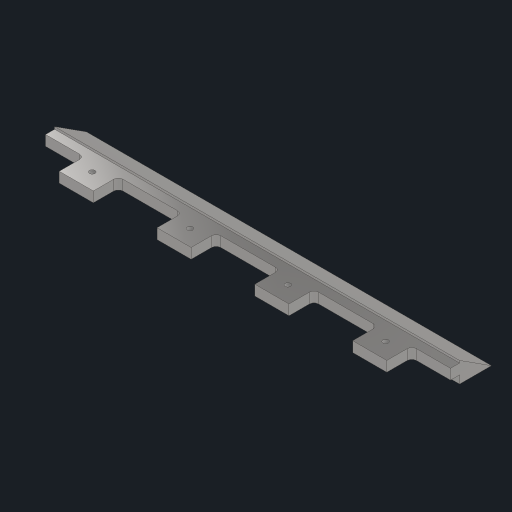
# Autodesk Inventor part: plog
Saved by Autodesk Inventor 2023 (Build 270158000, 158)
## iProperties
Created: 2024-04-10
Part Number: plog
Material: Steel, Alloy
Document SubType Name: Modeling
Designer: szymo
Density: 7.73 g/cm^3
Appearance: Semi-Polished
Mass: 132.729 g
Surface Area: 104.354 cm^2
Volume: 17.1707 cm^3
Author: szymo
Autodesk Inventor part; units mm, degrees
ref_plane "YZ Plane" through (0, 0, 0) normal (1, 0, 0) x (0, 1, 0)
ref_plane "XZ Plane" through (0, 0, 0) normal (0, 1, 0) x (-1, 0, 0)
ref_plane "XY Plane" through (0, 0, 0) normal (0, 0, 1) x (1, 0, 0)
sketch "Sketch3" plane through (0, 0, 0) normal (1, 0, 0) x (0, 1, 0)
  line L0 (0, 0) -> (9, 0)
  line L1 (9, 0) -> (9, -14)
  line L2 (9, -14) -> (0, -14)
  line L3 (0, -14) -> (0, 0)
  line L4 (9, 0) -> (0, -14)
  line L5 (8, 0) -> (3.5, 0)
  line L6 (3.5, 0) -> (3.5, 15)
  line L7 (3.5, 15) -> (8, 15)
  line L8 (8, 15) -> (8, 0)
  line L9 (8.5, 0) -> (8, 0)
  line L10 (8, 0) -> (8, 4)
  point P0 (3.5, 0)
  dimension "d30" = 15
  dimension "d31" = 4.5
  dimension "d63" = 9
  dimension "d141" = 32.735
  dimension "d142" = 14
  dimension "d143" = 3.5
  dimension "d144" = 1
  constraints: 22 end point, 4 perpendicular, 3 point on line, 1 collinear
  measures "d30" distance of L5.end L6.end
  measures "d31" distance of L6.end L7.end
  measures "d63" distance of L1.end L2.end
  measures "d141" angle of L4 L3
  measures "d142" distance of L0.end L1.end
  measures "d143" distance between parallel lines of L6 L3
  measures "d144" distance from line of L8 L0.end
extrude "Extrusion2" add sketch "Sketch3" along normal blind 178 contours L0 L4 L3 | L6 L7 L8 L0
sketch "Sketch10" plane through (0, 3.5, -14) normal (0, -1, 0) x (1, 0, 0)
  line L0 (0, 14) -> (0, 26)
  line L1 (0, 26) -> (178, 26)
  line L2 (178, 14) -> (178, 26)
  line L3 (0, 14) -> (0, 18)
  line L4 (0, 18) -> (17, 18)
  line L5 (17, 18) -> (17, 26)
  line L6 (17, 26) -> (0, 26)
  line L7 (0, 26) -> (0, 18)
  line L8 (0, 18) -> (178, 18)
  line L9 (178, 26) -> (161, 26)
  line L10 (161, 26) -> (161, 18)
  line L11 (161, 18) -> (178, 18)
  line L12 (178, 18) -> (178, 26)
  line L13 (17, 26) -> (32, 26)
  line L14 (32, 26) -> (32, 18)
  line L15 (32, 18) -> (17, 18)
  line L16 (17, 18) -> (17, 26)
  line L17 (60, 26) -> (75, 26)
  line L18 (75, 26) -> (75, 18)
  line L19 (75, 18) -> (60, 18)
  line L20 (60, 18) -> (60, 26)
  line L21 (103, 26) -> (118, 26)
  line L22 (118, 26) -> (118, 18)
  line L23 (118, 18) -> (103, 18)
  line L24 (103, 18) -> (103, 26)
  line L25 (146, 26) -> (161, 26)
  line L26 (161, 26) -> (161, 18)
  line L27 (161, 18) -> (146, 18)
  line L28 (146, 18) -> (146, 26)
  line L29 (17, 26) -> (32, 18)
  line L30 (32, 26) -> (17, 18)
  line L31 (60, 26) -> (75, 18)
  line L32 (75, 26) -> (60, 18)
  line L33 (103, 26) -> (118, 18)
  line L34 (118, 26) -> (103, 18)
  line L35 (146, 26) -> (161, 18)
  line L36 (161, 26) -> (146, 18)
  line L37 (0, 14) -> (178, 14)
  line L38 (178, 26) -> (161, 26)
  line L39 (161, 26) -> (161, 33.1494)
  line L40 (161, 33.1494) -> (178, 33.1494)
  line L41 (178, 33.1494) -> (178, 26)
  line L42 (146, 26) -> (118, 26)
  line L43 (118, 26) -> (118, 37.5544)
  line L44 (118, 37.5544) -> (146, 37.5544)
  line L45 (146, 37.5544) -> (146, 26)
  line L46 (103, 26) -> (75, 26)
  line L47 (75, 26) -> (75, 36.0625)
  line L48 (75, 36.0625) -> (103, 36.0625)
  line L49 (103, 36.0625) -> (103, 26)
  line L50 (60, 26) -> (32, 26)
  line L51 (32, 26) -> (32, 34.4304)
  line L52 (32, 34.4304) -> (60, 34.4304)
  line L53 (60, 34.4304) -> (60, 26)
  line L54 (17, 26) -> (0, 26)
  line L55 (0, 26) -> (0, 37.0756)
  line L56 (0, 37.0756) -> (17, 37.0756)
  line L57 (17, 37.0756) -> (17, 26)
  point P0 (118, 26)
  point P1 (24.5, 22)
  point P2 (67.5, 22)
  point P3 (110.5, 22)
  point P4 (153.5, 22)
  dimension "d118" = 17
  dimension "d119" = 17
  dimension "d120" = 15
  dimension "d121" = 15
  dimension "d122" = 15
  dimension "d123" = 15
  dimension "d124" = 0
  dimension "d125" = 0
  dimension "d126" = 28
  dimension "d129" = 28
  dimension "d130" = 28
  constraints: 116 end point, 10 parallel, 5 horizontal, 5 perpendicular, 5 point on line, 4 midpoint
  measures "d118" distance of L6.end L5.end
  measures "d119" distance of L11.end L10.end
  measures "d120" distance of L14.end L15.end
  measures "d121" distance of L18.end L19.end
  measures "d122" distance of L22.end L23.end
  measures "d123" distance of L26.end L27.end
  measures "d124" distance between parallel lines of L5 L16
  measures "d125" distance between parallel lines of L26 L10
  measures "d126" distance between parallel lines of L22 L28
  measures "d129" distance between parallel lines of L14 L20
  measures "d130" distance between parallel lines of L18 L24
extrude "Extrusion5" cut sketch "Sketch10" against normal up to next contours L0 L1 L5 L4 | L55 L56 L57 L1 | L8 L10 L1 L2 | L14 L1 L20 L8 | L1 L39 L40 L41 | L51 L52 L53 L1 | L8 L22 L1 L28 | L18 L1 L24 L8 | L1 L43 L44 L45 | L47 L48 L49 L1
fillet "Fillet3" radius 2 8 edges at (161, 5.75, 4) (146, 5.75, 4) (118, 5.75, 4) (103, 5.75, 4) (75, 5.75, 4) (60, 5.75, 4) (32, 5.75, 4) (17, 5.75, 4)
sketch "Sketch11" plane through (0, 8, 0) normal (0, 1, 0) x (1, 0, 0)
  point P0 (0, 0)
  point P1 (24.5, -8)
  point P2 (67.5, -8)
  point P3 (110.5, -8)
  point P4 (153.5, -8)
hole "Hole5" at (24.5, 8, 8) at (67.5, 8, 8) at (110.5, 8, 8) at (153.5, 8, 8) direction (0, -1, 0) diameter 2.459 depth 8.8 thread size "M3x0.5" class "6H" standard "ISO Metric profile"
equation "\"d126\" = d130"
equation "\"d129\" = d130"
body "Solid2"
